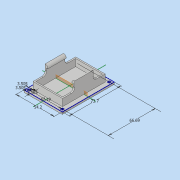
# Autodesk Inventor part: esc_holder
Saved by Autodesk Inventor 2017 (Build 210142000, 142)
## iProperties
Created: 2017-02-25
Part Number: esc_holder
Material: Generic
Document SubType Name: Modeling
Designer: Joshua Yuan
Density: 1 g/cm^3
Appearance: Default
Author: Joshua Yuan
Autodesk Inventor part; units mm, degrees
ref_plane "YZ Plane" through (0, 0, 0) normal (1, 0, 0) x (0, 1, 0)
ref_plane "XZ Plane" through (0, 0, 0) normal (0, 1, 0) x (-1, 0, 0)
ref_plane "XY Plane" through (0, 0, 0) normal (0, 0, 1) x (1, 0, 0)
sketch "Sketch1" plane through (0, 0, 0) normal (0, 1, 0) x (-1, 0, 0)
  line L0 (27.1, 36.85) -> (-27.1, 36.85)
  line L1 (-27.1, 36.85) -> (-27.1, -36.85)
  line L2 (-27.1, -36.85) -> (27.1, -36.85)
  line L3 (27.1, -36.85) -> (27.1, 36.85)
  line L4 (37.94, 0) -> (-37.94, 0) projected
  line L5 (0, -51.59) -> (0, 51.59) projected
  circle A0 centre (23.5948, 33.3448) radius 1.7526
  circle A1 centre (-23.5952, 33.3448) radius 1.7526
  circle A2 centre (23.5948, -33.3452) radius 1.7526
  circle A3 centre (-23.5952, -33.3452) radius 1.7526
  point P0 (0, 0)
  dimension "d0" = 54.2
  dimension "d1" = 73.7
  dimension "d16" = 3.5052
  dimension "d17" = 3.5052
  dimension "d18" = 3.5052
  dimension "d21" = 47.19
  dimension "d24" = 66.69
  constraints: 8 end point, 4 centre point, 2 horizontal, 2 parallel, 1 perpendicular, 1 vertical, 8 other
  measures "d0" distance of L0.start L0.end
  measures "d1" distance of L0.end L1.end
  measures "d16" diameter of A0
  measures "d17" distance from line of L0 A0.centre
  measures "d18" distance from line of L3 A0.centre
  measures "d21" distance of A0.centre A1.centre
  measures "d24" distance of A0.centre A2.centre
extrude "baseplate" add sketch "Sketch1" against normal blind 3.175 contours L3 L4 L5 L0 | L5 L4 L1 L0 | L3 L2 L5 L4 | L5 L2 L1 L4 | A0 | A1 | A2 | A3
sketch "Sketch2" plane through (0, 0, 0) normal (0, 1, 0) x (1, 0, 0)
  line L0 (19, 28.25) -> (-19, 28.25)
  line L1 (-19, 28.25) -> (-19, -28.25)
  line L2 (-19, -28.25) -> (19, -28.25)
  line L3 (19, -28.25) -> (19, 28.25)
  line L4 (-37.94, 0) -> (37.94, 0) projected
  line L5 (0, 51.59) -> (0, -51.59) projected
  line L6 (-21, -30.25) -> (-21, 30.25)
  line L7 (-21, 30.25) -> (21, 30.25)
  line L8 (21, 30.25) -> (21, -30.25)
  line L9 (21, -30.25) -> (-21, -30.25)
  dimension "d4" = 38
  dimension "d5" = 56.5
  dimension "d6" = 2
  constraints: 16 end point, 4 parallel, 2 perpendicular, 1 horizontal, 5 other
  measures "d4" distance of L1.end L2.end
  measures "d5" distance of L2.end L0.start
  measures "d6" distance between parallel lines of L1 L6
extrude "perimeter" add sketch "Sketch2" along normal blind 10 contours L0 L5 L7 L8 L4 L3 | L0 L1 L4 L6 L7 L5 | L4 L8 L9 L5 L2 L3 | L1 L2 L5 L9 L6 L4
ref_plane "Work Plane1" through (-27.1, 0, 0) normal (0, 0, 1) x (1, 0, 0)
sketch "Sketch3" plane through (-27.1, 0, 0) normal (0, 0, 1) x (1, 0, 0)
  line L0 (48.1, 10) -> (46.1, 10)
  line L1 (46.1, 10) -> (46.1, 19)
  line L2 (46.1, 19) -> (44.1, 19)
  line L3 (48.1, 10) -> (48.1, 23)
  arc A0 (48.1, 23) -> (44.1, 19) centre (48.1, 19) ccw
  line L4 (27.1, 0) -> (27.1, 45.1965)
  line L5 (6.1, 10) -> (8.1, 10)
  line L6 (8.1, 10) -> (8.1, 19)
  line L7 (8.1, 19) -> (10.1, 19)
  line L8 (6.1, 10) -> (6.1, 23)
  arc A1 (10.1, 19) -> (6.1, 23) centre (6.1, 19) ccw
  dimension "d10" = 2
  dimension "d11" = 2
  dimension "d12" = 9
  dimension "d13" = 13
  constraints: 18 end point, 6 symmetric about line, 4 point on circle, 2 centre point, 2 perpendicular, 2 vertical, 1 horizontal, 1 point on line, 1 other
  measures "d10" distance of L1.end L2.end
  measures "d11" distance of L0.start L0.end
  measures "d12" distance of L0.end L1.end
  measures "d13" distance of L0.start L3.end
extrude "holders" add sketch "Sketch3" along normal mid plane 26
extrude "Extrusion4" cut sketch "Sketch1" against normal blind 10 contours A0 | A1 | A2 | A3
fillet "Fillet1" radius 5 4 edges at (20, 10, -13) (-20, 10, -13) (20, 10, 13) (-20, 10, 13)
body "Solid1"
